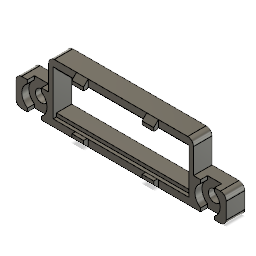
5v_psupply_mount (Autodesk Fusion 360 design; units mm, degrees)
Autodesk Fusion 360 part; units mm, degrees
sketch "Sketch1" plane through (0, 0, 0) normal (0, 0, 1) x (1, 0, 0)
  line L0 (0, 0) -> (12, 0)
  line L1 (12, 0) -> (12, 90)
  line L2 (12, 90) -> (0, 90)
  line L3 (0, 0) -> (0, 14)
  line L4 (0, 14) -> (-13.25, 14)
  line L5 (-13.25, 14) -> (-13.25, 76)
  line L6 (-13.25, 76) -> (0, 76)
  line L7 (0, 76) -> (0, 90)
  line L8 (-10.25, 74) -> (9, 74)
  line L9 (9, 74) -> (9, 16)
  line L10 (9, 16) -> (-10.25, 16)
  line L11 (-10.25, 16) -> (-10.25, 74)
  line L12 (9, 45) -> (12, 45) construction
  line L13 (-13.25, 45) -> (-10.25, 45) construction
  line L14 (-2.6313, 76) -> (-2.6313, 74) construction
  line L15 (12, 45) -> (6, 45) construction
  line L16 (6, 45) -> (6, 8) construction
  line L17 (6, 45) -> (6, 82) construction
  line L18 (6, 90) -> (6, 82) construction
  circle A0 centre (6, 82) radius 2.6
  circle A1 centre (6, 8) radius 2.6
  circle A2 centre (6, 82) radius 5.4
  circle A3 centre (6, 8) radius 5.4
  line L19 (-8.0045, 85) -> (29, 85)
  line L20 (29, 85) -> (29, 79)
  line L21 (29, 79) -> (-8.0045, 79)
  line L22 (-8.0045, 79) -> (-8.0045, 85)
  line L23 (6, 82) -> (-8.0045, 82) construction
  line L24 (-6, 11) -> (49, 11)
  line L25 (49, 11) -> (49, 5)
  line L26 (49, 5) -> (-6, 5)
  line L27 (-6, 5) -> (-6, 11)
  line L28 (6, 8) -> (-6, 8) construction
  dimension "d1" = 90
  dimension "d2" = 12
  dimension "d3" = 58
  dimension "d4" = 19.25
  dimension "d5" = 2
  dimension "d6" = 8
  dimension "d7" = 5.2
  dimension "d8" = 10.8
  dimension "d9" = 3
  dimension "d10" = 6
  dimension "d11" = 6
  measures "d2" distance of L0.start
  measures "d7" diameter of A1
  measures "d8" diameter of A2
extrude "Extrude1" add sketch "Sketch1" against normal blind 8 contours L0 L1 L3 A3 L26 | L3 A3 L24 L26 | L1 A3 L24 L26 | L1 L3 L4 L5 L6 L7 A2 A3 L21 L24 | A3 L26 | A3 L24 L26 | A3 L24 | L1 A2 L19 L21 | L1 L2 L7 A2 L19 | A2 L19 L21 | A2 L21 | A2 L19 | L7 A2 L19 L21 | L8 L9 L10 L11
extrude "Extrude2" cut sketch "Sketch1" against normal blind 3 contours L3 A3 L24 L26 | L1 A3 L24 L26 | A3 L26 | A3 L24 L26 | A3 L24 | L1 A2 L19 L21 | A2 L19 L21 | A2 L21 | A2 L19 | L7 A2 L19 L21
extrude "Extrude3" cut sketch "Sketch1" against normal blind 1.4 contours L8 L9 L10 L11
fillet "Fillet1" radius 2.5 6 edges at (0, 90, -4) (12, 90, -4) (0, 0, -4) (12, 0, -4) (-13.25, 14, -4) (-13.25, 76, -4)
sketch "Sketch2" plane through (0, 0, -1.4) normal (0, 0, 1) x (1, 0, 0)
  line L0 (-10.25, 16) -> (9, 16)
  line L1 (9, 16) -> (9, 74)
  line L2 (9, 74) -> (-10.25, 74)
  line L3 (-10.25, 74) -> (-10.25, 16)
  line L4 (-8.725, 74) -> (7.475, 74)
  line L5 (7.475, 74) -> (7.475, 16)
  line L6 (7.475, 16) -> (-8.725, 16)
  line L7 (-8.725, 16) -> (-8.725, 74)
  line L8 (-8.725, 45) -> (-10.25, 45) construction
  line L9 (7.475, 45) -> (9, 45) construction
  dimension "d19" = 16.2
  dimension "d20" = 58
extrude "Extrude4" cut sketch "Sketch2" against normal blind 29 contours L0 L2 L4 L5 L6 L7
sketch "Sketch3" plane through (0, 14, 0) normal (0, -1, 0) x (1, 0, 0)
  line L0 (-10.75, 0) -> (-10.75, -8)
  line L1 (-10.75, -8) -> (0, -8)
  line L2 (0, -8) -> (0, 0)
  line L3 (0, 0) -> (-10.75, 0)
  line L4 (-13.25, 0) -> (-13.25, 2)
  line L5 (-13.25, 2) -> (-9.75, 2)
  line L6 (-9.75, 2) -> (-9.75, 0.5)
  line L7 (-9.75, 0.5) -> (-10.25, 0)
  line L8 (-10.25, 0) -> (-13.25, 0)
  line L9 (12, 0) -> (12, -8)
  line L10 (12, 0) -> (12, 2)
  line L11 (12, 2) -> (8.5, 2)
  line L12 (8.5, 2) -> (8.5, 0.5)
  line L13 (8.5, 0.5) -> (9, 0)
  line L14 (9, 0) -> (12, 0)
  dimension "d23" = 3.5
  dimension "d26" = 3
  dimension "d27" = 1.5
  dimension "d28" = 2
  dimension "d29" = 3.5
  dimension "d30" = 2
  dimension "d31" = 1.5
  dimension "d41" = 3
extrude "Extrude5" add sketch "Sketch3" against normal blind 64 contours L3 L4 L5 L6 L7 L8 | L10 L11 L12 L13 L14
sketch "Sketch4" plane through (0, 0, 2) normal (0, 0, 1) x (1, 0, 0)
  line L0 (-13.25, 14) -> (-9.75, 14)
  line L1 (-9.75, 14) -> (-9.75, 78)
  line L2 (-9.75, 78) -> (-13.25, 78)
  line L3 (-13.25, 78) -> (-13.25, 14)
  line L4 (-43, 87) -> (35, 87)
  line L5 (35, 87) -> (35, 61)
  line L6 (35, 61) -> (-43, 61)
  line L7 (-43, 61) -> (-43, 87)
  line L8 (-33, 56) -> (44, 56)
  line L9 (44, 56) -> (44, 31)
  line L10 (44, 31) -> (-33, 31)
  line L11 (-33, 31) -> (-33, 56)
  line L12 (-33, 26) -> (46, 26)
  line L13 (46, 26) -> (46, 6)
  line L14 (46, 6) -> (-33, 6)
  line L15 (-33, 6) -> (-33, 26)
  line L16 (-23, 61) -> (-23, 56) construction
  line L17 (-27, 31) -> (-27, 26) construction
  line L18 (9, 16) -> (-10.25, 16)
  line L19 (-5.0331, 26) -> (-5.0331, 16) construction
  line L20 (-10.25, 74) -> (9, 74)
  line L21 (-6, 61) -> (-6, 74) construction
  dimension "d36" = 5
  dimension "d37" = 5
  dimension "d38" = 10
  dimension "d39" = 13
extrude "Extrude6" cut sketch "Sketch4" against normal blind 2 contours L0 L1 L3 L12 | L0 L1 L3 L12 L13 L14 L15 | L3 L8 L10 L11 | L1 L3 L8 L10 | L1 L8 L9 L10 | L1 L2 L3 L4 L5 L6 L7 | L1 L2 L3 L6
chamfer "Chamfer1" distance 2 angle 45 4 edges at (12, 58.5, 2) (-13.25, 58.5, 2) (-13.25, 28.5, 2) (12, 28.5, 2)
move_body "Move1" bodies 1 to x (0, -1, 0) y (1, 0, 0) z (0, 0, 1) at (-13.25, -13.25, 0)
